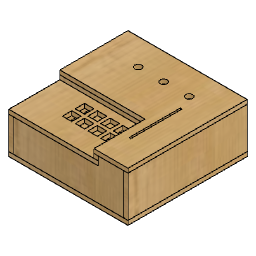
MIDI Mixer v3 (Autodesk Fusion 360 design; units mm, degrees)
Autodesk Fusion 360 part; units mm, degrees
sketch "Sketch1" plane through (0, 0, 0) normal (0, 0, 1) x (1, 0, 0)
  line L0 (0, 0) -> (100, 0) construction
  line L1 (100, 0) -> (100, 100) construction
  line L2 (100, 100) -> (0, 100) construction
  line L3 (0, 100) -> (0, 0) construction
  line L4 (120, -20) -> (-20, -20)
  line L5 (-20, -20) -> (-20, 120)
  line L6 (-20, 120) -> (120, 120)
  line L7 (120, 120) -> (120, -20)
  line L8 (100, 0) -> (95, 0) construction
  line L9 (95, 0) -> (95, 12) construction
  line L10 (95, 12) -> (100, 12) construction
  line L11 (100, 12) -> (100, 0) construction
  line L12 (95, 12) -> (86, 12) construction
  line L13 (86, 12) -> (86, 72) construction
  line L14 (86, 72) -> (95, 72) construction
  line L15 (95, 72) -> (95, 12) construction
  line L16 (90.5, 72) -> (90.5, 12)
  line L17 (91.5, 72) -> (89.5, 72)
  line L18 (89.5, 72) -> (89.5, 12)
  line L19 (89.5, 12) -> (91.5, 12)
  line L20 (91.5, 12) -> (91.5, 72)
  line L21 (91.5, 72) -> (89.5, 12) construction
  line L22 (89.5, 72) -> (91.5, 12) construction
  line L23 (0, 100) -> (23, 100) construction
  line L24 (23, 100) -> (23, 89) construction
  line L25 (23, 89) -> (0, 89) construction
  line L26 (0, 89) -> (0, 100) construction
  circle A0 centre (23, 89) radius 4
  line L27 (23, 89) -> (53, 89) construction
  line L28 (53, 89) -> (83, 89) construction
  circle A1 centre (53, 89) radius 4
  circle A2 centre (83, 89) radius 4
  line L29 (0, 0) -> (24, 0) construction
  line L30 (24, 0) -> (24, 10) construction
  line L31 (24, 10) -> (0, 10) construction
  line L32 (0, 10) -> (0, 0) construction
  line L33 (29.5, 15.5) -> (18.5, 15.5)
  line L34 (18.5, 15.5) -> (18.5, 4.5)
  line L35 (18.5, 4.5) -> (29.5, 4.5)
  line L36 (29.5, 4.5) -> (29.5, 15.5)
  line L37 (29.5, 15.5) -> (18.5, 4.5) construction
  line L38 (18.5, 15.5) -> (29.5, 4.5) construction
  line L39 (44.5, 15.5) -> (33.5, 15.5)
  line L40 (44.5, 4.5) -> (44.5, 15.5)
  line L41 (33.5, 4.5) -> (44.5, 4.5)
  line L42 (33.5, 15.5) -> (33.5, 4.5)
  line L43 (59.5, 15.5) -> (48.5, 15.5)
  line L44 (59.5, 4.5) -> (59.5, 15.5)
  line L45 (48.5, 4.5) -> (59.5, 4.5)
  line L46 (48.5, 15.5) -> (48.5, 4.5)
  line L47 (74.5, 15.5) -> (63.5, 15.5)
  line L48 (74.5, 4.5) -> (74.5, 15.5)
  line L49 (63.5, 4.5) -> (74.5, 4.5)
  line L50 (63.5, 15.5) -> (63.5, 4.5)
  line L51 (18.5, 30.5) -> (29.5, 19.5) construction
  line L52 (44.5, 30.5) -> (33.5, 30.5)
  line L53 (48.5, 19.5) -> (59.5, 19.5)
  line L54 (74.5, 30.5) -> (63.5, 30.5)
  line L55 (63.5, 19.5) -> (74.5, 19.5)
  line L56 (44.5, 19.5) -> (44.5, 30.5)
  line L57 (48.5, 30.5) -> (48.5, 19.5)
  line L58 (18.5, 19.5) -> (29.5, 19.5)
  line L59 (29.5, 19.5) -> (29.5, 30.5)
  line L60 (18.5, 30.5) -> (18.5, 19.5)
  line L61 (33.5, 19.5) -> (44.5, 19.5)
  line L62 (29.5, 30.5) -> (18.5, 30.5)
  line L63 (59.5, 19.5) -> (59.5, 30.5)
  line L64 (29.5, 30.5) -> (18.5, 19.5) construction
  line L65 (33.5, 30.5) -> (33.5, 19.5)
  line L66 (74.5, 19.5) -> (74.5, 30.5)
  line L67 (63.5, 30.5) -> (63.5, 19.5)
  line L68 (59.5, 30.5) -> (48.5, 30.5)
  line L69 (-20, 40) -> (85, 40)
  line L70 (85, 40) -> (85, 45)
  line L71 (85, 45) -> (-20, 45)
  line L72 (-20, 45) -> (-20, 40)
  line L73 (85, 40) -> (80, 40)
  line L74 (80, 40) -> (80, -20)
  line L75 (80, -20) -> (85, -20)
  line L76 (85, -20) -> (85, 40)
  point P0 (50, 50)
  point P1 (90.5, 42)
  point P2 (24, 10)
  point P3 (24, 25)
  point P4 (24, 25)
  dimension "d1" = 100
  dimension "d2" = 100
  dimension "d3" = 140
  dimension "d4" = 140
  dimension "d5" = 5
  dimension "d6" = 12
  dimension "d7" = 9
  dimension "d8" = 60
  dimension "d9" = 2
  dimension "d10" = 60
  dimension "d11" = 23
  dimension "d12" = 11
  dimension "d13" = 8
  dimension "d14" = 30
  dimension "d15" = 30
  dimension "d16" = 8
  dimension "d17" = 8
  dimension "d18" = 24
  dimension "d19" = 10
  dimension "d20" = 11
  dimension "d21" = 11
  dimension "d24" = 45
  dimension "d25" = 0
  dimension "d28" = 0
  dimension "d29" = 15
  dimension "d30" = 105
  dimension "d31" = 5
  dimension "d32" = 5
  constraint horizontal L0
  constraint vertical L1
  constraint horizontal L2
  constraint vertical L3
  constraint coincident L0.start L3.end
  constraint horizontal L4
  constraint perpendicular L4 L5
  constraint parallel L4 L6
  constraint parallel L5 L7
  constraint horizontal L8
  constraint vertical L9
  constraint horizontal L10
  constraint vertical L11
  constraint horizontal L12
  constraint vertical L13
  constraint horizontal L14
  constraint vertical L15
  constraint midpoint L14 L16.start
  constraint midpoint L12 L16.end
  constraint horizontal L17
  constraint perpendicular L17 L18
  constraint parallel L17 L19
  constraint parallel L18 L20
  constraint coincident L21 P1
  constraint coincident L22 P1
  constraint midpoint L16 P1
  constraint horizontal L23
  constraint vertical L24
  constraint horizontal L25
  constraint vertical L26
  constraint coincident L24.end L25.start
  constraint perpendicular L24 L27
  constraint parallel L27 L28
  constraint coincident L27.end L28.start
  constraint coincident L28.end A2.centre
  constraint horizontal L29
  constraint vertical L30
  constraint horizontal L31
  constraint vertical L32
  constraint horizontal L33
  constraint perpendicular L33 L34
  constraint parallel L33 L35
  constraint parallel L34 L36
  constraint coincident L37 P2
  constraint coincident L38 P2
  constraint coincident P2 L30.end
  constraint horizontal L69
  constraint vertical L70
  constraint horizontal L71
  constraint vertical L72
  constraint coincident L5 L69.start
  constraint horizontal L73
  constraint vertical L74
  constraint horizontal L75
  constraint vertical L76
  measures "d1" distance of L0.start L0.end
  measures "d2" distance of L0.start L2.end
  measures "d3" distance of L5.end L6.end
  measures "d4" distance of L4.end L5.end
  measures "d5" distance of L0.end L8.end
  measures "d6" distance of L0.end L10.end
  measures "d7" distance of L9.end L12.end
  measures "d8" distance of L9.end L14.end
  measures "d9" distance of L18.end L19.end
  measures "d10" distance of L17.end L18.end
  measures "d11" distance of L2.end L23.end
  measures "d12" distance of L2.end L25.end
  measures "d13" diameter of A0
  measures "d14" distance of L24.end L27.end
  measures "d15" distance of L27.end L28.end
  measures "d16" diameter of A1
  measures "d17" diameter of A2
  measures "d18" distance of L0.start L29.end
  measures "d19" distance of L0.start L31.end
  measures "d20" distance of L34.end L35.end
  measures "d21" distance of L33.end L34.end
  measures "d30" distance of L69.start L69.end
  measures "d31" distance of L69.start L71.end
  measures "d32" distance of L69.end L73.end
extrude "Extrude1" add sketch "Sketch1" along normal blind 5 contours L4 L5 L6 L7 L70 L71 L76 | L4 L69 L73 L74 L75 L76 | L5 L69 L70 L71 L72 L73 makes body 1
extrude "Extrude2" add sketch "Sketch1" along normal blind 5 separate body contours L4 L69 L73 L74 L75 L76 | L4 L5 L69 L74 | L5 L69 L70 L71 L72 L73 makes body 2
move_body "Move1" bodies 2 to x (1, 0, 0) y (0, 1, 0) z (0, 0, 1) at (0, 0, -10)
extrude "Extrude3" add sketch "Sketch1" against normal blind 5 separate body contours L4 L69 L73 L74 L75 L76 | L5 L69 L70 L71 L72 L73 makes body 3
sketch "Sketch2" plane through (-20, 0, 0) normal (-1, 0, 0) x (0, -1, 0)
  line L0 (-120, 0) -> (-40, 0)
  line L1 (-40, 0) -> (-40, 5)
  line L2 (-40, 5) -> (-120, 5)
  line L3 (-120, 5) -> (-120, 0)
  line L4 (-120, 0) -> (-45, 0)
  line L5 (-45, 0) -> (-45, -10)
  line L6 (-45, -10) -> (20, -10)
  line L7 (20, -10) -> (20, -48.1)
  line L8 (20, -48.1) -> (-120, -48.1)
  line L9 (-120, -48.1) -> (-120, 0)
  dimension "d39" = 38.1
  constraint coincident L0.start L3.end
  constraint coincident L0 L4.end
  constraint perpendicular L3 L4
  constraint perpendicular L4 L5
  constraint perpendicular L5 L6
  constraint perpendicular L6 L7
  constraint perpendicular L3 L8
  constraint perpendicular L0 L9
  measures "d39" distance of L6.end L7.end
extrude "Extrude4" add sketch "Sketch2" against normal blind 5 separate body contours L0 L4 L5 L6 L7 L8 L9 makes body 4
sketch "Sketch3" plane through (120, 0, 0) normal (1, 0, 0) x (0, 1, 0)
  line L0 (-20, 0) -> (120, 0)
  line L1 (120, 0) -> (120, 5)
  line L2 (120, 5) -> (-20, 5)
  line L3 (-20, 5) -> (-20, 0)
  line L4 (-20, -48.1) -> (120, -48.1)
  line L5 (120, -48.1) -> (120, 0)
  line L6 (120, 0) -> (45, 0)
  line L7 (45, 0) -> (45, -10)
  line L8 (45, -10) -> (-20, -10)
  line L9 (-20, -10) -> (-20, -48.1)
  line L10 (-20, -10) -> (-20, 0)
  line L11 (45, 0) -> (-20, 0)
  constraint coincident L8.end L9.start
  constraint coincident L0.start L3.end
  constraint coincident L6.end L7.start
extrude "Extrude5" add sketch "Sketch3" against normal blind 5 separate body contours L0 L7 L8 L10 L11 | L0 L4 L5 L6 L7 L8 L9 makes body 5
sketch "Sketch4" plane through (0, -20, 0) normal (0, -1, 0) x (1, 0, 0)
  line L0 (-20, -10) -> (85, -10)
  line L1 (85, -10) -> (85, -5)
  line L2 (85, -5) -> (-20, -5)
  line L3 (-20, -5) -> (-20, -10)
  line L4 (-20, -10) -> (85, -10)
  line L5 (85, -10) -> (85, -5)
  line L6 (85, 0) -> (85, -5)
  line L7 (80, 0) -> (120, 0)
  line L8 (115, -48.1) -> (115, 0)
  line L9 (-15, -10) -> (-15, -48.1)
  line L10 (115, -48.1) -> (-15, -48.1)
  constraint coincident L8.start L10.start
  constraint coincident L9.end L10.end
extrude "Extrude6" add sketch "Sketch4" against normal blind 5 separate body contours L0 L1 L4 L5 L6 L7 L8 L9 L10 makes body 6
sketch "Sketch5" plane through (0, 120, 0) normal (0, 1, 0) x (-1, 0, 0)
  line L0 (-120, 0) -> (20, 0)
  line L1 (20, 0) -> (20, 5)
  line L2 (20, 5) -> (-120, 5)
  line L3 (-120, 5) -> (-120, 0)
  line L4 (-115, 0) -> (-115, -48.1)
  line L5 (20, 0) -> (-120, 0)
  line L6 (15, -48.1) -> (15, 0)
  line L7 (-115, -48.1) -> (15, -48.1)
  constraint coincident L4.end L7.start
  constraint coincident L6.start L7.end
extrude "Extrude7" add sketch "Sketch5" against normal blind 5 separate body contours L0 L4 L5 L6 L7 makes body 7
sketch "Sketch6" plane through (0, 0, -48.1) normal (0, 0, -1) x (1, 0, 0)
  line L0 (-20, 20) -> (-20, -120)
  line L1 (-20, -120) -> (-15, -120)
  line L2 (-15, -120) -> (-15, 20)
  line L3 (-15, 20) -> (-20, 20)
  line L4 (-20, 20) -> (-20, -120)
  line L5 (115, 20) -> (-15, 20)
  line L6 (-20, 20) -> (-15, 20)
  line L7 (120, 20) -> (115, 20)
  line L8 (120, 20) -> (120, -120)
  line L9 (120, -120) -> (115, -120)
  line L10 (115, -120) -> (-15, -120)
  line L11 (-20, -120) -> (-15, -120)
extrude "Extrude8" add sketch "Sketch6" along normal blind 5 separate body makes body 8
sketch "Sketch7" plane through (-20, 0, 0) normal (-1, 0, 0) x (0, -1, 0)
  line L0 (-120, -48.1) -> (20, -48.1)
  line L1 (20, -48.1) -> (20, -10)
  line L2 (20, -10) -> (-45, -10)
  line L3 (-45, -10) -> (-45, 0)
  line L4 (-45, 0) -> (-120, 0)
  line L5 (-120, 0) -> (-120, -48.1)
  line L6 (-100, 0) -> (0, 0)
  line L7 (-100, 0) -> (-67, 0) construction
  line L8 (-67, 0) -> (-67, -15) construction
  line L9 (-67, -15) -> (-100, -15) construction
  line L10 (-100, -15) -> (-100, 0) construction
  line L11 (-67, -15) -> (-57, -15)
  line L12 (-57, -15) -> (-57, -25)
  line L13 (-57, -25) -> (-67, -25)
  line L14 (-67, -25) -> (-67, -15)
  dimension "d50" = 33
  dimension "d51" = 15
  dimension "d52" = 10
  dimension "d53" = 10
  constraint horizontal L7
  constraint vertical L8
  constraint horizontal L9
  constraint vertical L10
  constraint coincident L6.start L7.start
  constraint horizontal L11
  constraint vertical L12
  constraint horizontal L13
  constraint vertical L14
  measures "d50" distance of L6.start L7.end
  measures "d51" distance of L6.start L9.end
  measures "d52" distance of L8.end L11.end
  measures "d53" distance of L8.end L13.end
extrude "Extrude9" cut sketch "Sketch7" against normal blind 9 contours L11 L12 L13 L14 bodies 4
sketch "topTop" plane through (0, 0, 5) normal (0, 0, 1) x (-1, 0, 0)
  circle A0 centre (-83, -89) radius 4
  circle A1 centre (-53, -89) radius 4
  circle A2 centre (-23, -89) radius 4
  line L0 (-91.5, -72) -> (-91.5, -12)
  line L1 (-91.5, -12) -> (-89.5, -12)
  line L2 (-89.5, -12) -> (-89.5, -72)
  line L3 (-89.5, -72) -> (-91.5, -72)
  line L4 (20, -120) -> (20, -40)
  line L5 (20, -40) -> (-80, -40)
  line L6 (-80, -40) -> (-80, 20)
  line L7 (-80, 20) -> (-120, 20)
  line L8 (-120, 20) -> (-120, -120)
  line L9 (-120, -120) -> (20, -120)
sketch "filler" plane through (0, 0, 0) normal (0, 0, 1) x (-1, 0, 0)
  line L0 (-85, 20) -> (-85, -45)
  line L1 (-85, -45) -> (20, -45)
  line L2 (20, -45) -> (20, -40)
  line L3 (20, -40) -> (-80, -40)
  line L4 (-80, -40) -> (-80, 20)
  line L5 (-80, 20) -> (-85, 20)
sketch "topBot" plane through (0, 0, -5) normal (0, 0, 1) x (-1, 0, 0)
  line L0 (-18.5, -30.5) -> (-29.5, -30.5)
  line L1 (-29.5, -30.5) -> (-29.5, -19.5)
  line L2 (-29.5, -19.5) -> (-18.5, -19.5)
  line L3 (-18.5, -19.5) -> (-18.5, -30.5)
  line L4 (-63.5, -4.5) -> (-63.5, -15.5)
  line L5 (-63.5, -15.5) -> (-74.5, -15.5)
  line L6 (-74.5, -15.5) -> (-74.5, -4.5)
  line L7 (-74.5, -4.5) -> (-63.5, -4.5)
  line L8 (-48.5, -4.5) -> (-48.5, -15.5)
  line L9 (-48.5, -15.5) -> (-59.5, -15.5)
  line L10 (-59.5, -15.5) -> (-59.5, -4.5)
  line L11 (-59.5, -4.5) -> (-48.5, -4.5)
  line L12 (-33.5, -4.5) -> (-33.5, -15.5)
  line L13 (-33.5, -15.5) -> (-44.5, -15.5)
  line L14 (-44.5, -15.5) -> (-44.5, -4.5)
  line L15 (-44.5, -4.5) -> (-33.5, -4.5)
  line L16 (-48.5, -30.5) -> (-59.5, -30.5)
  line L17 (-59.5, -30.5) -> (-59.5, -19.5)
  line L18 (-59.5, -19.5) -> (-48.5, -19.5)
  line L19 (-48.5, -19.5) -> (-48.5, -30.5)
  line L20 (-33.5, -19.5) -> (-33.5, -30.5)
  line L21 (-33.5, -30.5) -> (-44.5, -30.5)
  line L22 (-44.5, -30.5) -> (-44.5, -19.5)
  line L23 (-44.5, -19.5) -> (-33.5, -19.5)
  line L24 (-29.5, -15.5) -> (-29.5, -4.5)
  line L25 (-29.5, -4.5) -> (-18.5, -4.5)
  line L26 (-18.5, -4.5) -> (-18.5, -15.5)
  line L27 (-18.5, -15.5) -> (-29.5, -15.5)
  line L28 (-63.5, -19.5) -> (-63.5, -30.5)
  line L29 (-63.5, -30.5) -> (-74.5, -30.5)
  line L30 (-74.5, -30.5) -> (-74.5, -19.5)
  line L31 (-74.5, -19.5) -> (-63.5, -19.5)
  line L32 (20, 20) -> (-85, 20)
  line L33 (-85, 20) -> (-85, -45)
  line L34 (-85, -45) -> (20, -45)
  line L35 (20, -45) -> (20, 20)
sketch "rightSide" plane through (120, 0, 0) normal (1, 0, 0) x (0, 1, 0)
  line L0 (-20, 0) -> (-20, -48.1)
  line L1 (-20, -48.1) -> (120, -48.1)
  line L2 (120, -48.1) -> (120, 0)
  line L3 (120, 0) -> (-20, 0)
sketch "front" plane through (0, -20, 0) normal (0, -1, 0) x (1, 0, 0)
  line L0 (85, 0) -> (85, -10)
  line L1 (85, -10) -> (-15, -10)
  line L2 (-15, -10) -> (-15, -48.1)
  line L3 (-15, -48.1) -> (115, -48.1)
  line L4 (115, -48.1) -> (115, 0)
  line L5 (115, 0) -> (85, 0)
sketch "leftSide" plane through (-20, 0, 0) normal (-1, 0, 0) x (0, -1, 0)
  line L0 (-57, -15) -> (-57, -25)
  line L1 (-57, -25) -> (-67, -25)
  line L2 (-67, -25) -> (-67, -15)
  line L3 (-67, -15) -> (-57, -15)
  line L4 (-120, -48.1) -> (20, -48.1)
  line L5 (20, -48.1) -> (20, -10)
  line L6 (20, -10) -> (-45, -10)
  line L7 (-45, -10) -> (-45, 0)
  line L8 (-45, 0) -> (-120, 0)
  line L9 (-120, 0) -> (-120, -48.1)
sketch "back" plane through (0, 120, 0) normal (0, 1, 0) x (-1, 0, 0)
  line L0 (-115, -48.1) -> (15, -48.1)
  line L1 (15, -48.1) -> (15, 0)
  line L2 (15, 0) -> (-115, 0)
  line L3 (-115, 0) -> (-115, -48.1)
sketch "bottom" plane through (0, 0, -53.1) normal (0, 0, -1) x (1, 0, 0)
  line L0 (-20, 20) -> (-20, -120)
  line L1 (-20, -120) -> (120, -120)
  line L2 (120, -120) -> (120, 20)
  line L3 (120, 20) -> (-20, 20)
named bodies: "topTop", "topBot", "filler", "leftSide", "rightSide", "front", "back", "bottom"
